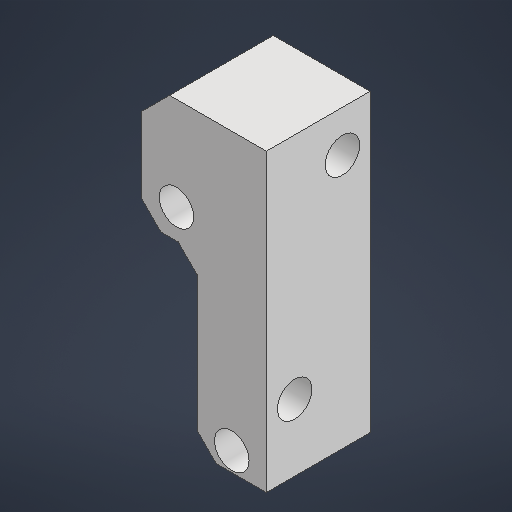
# Autodesk Inventor part: xy转接连杆
Saved by Autodesk Inventor 2025 (Build 290162000, 162)
## iProperties
Created: 2025-12-12
Part Number: xy转接连杆
Material: 常规
Document SubType Name: Modeling
Designer: HZD
Density: 1 g/cm^3
Appearance: 默认
Author: HZD
Autodesk Inventor part; units mm, degrees
ref_plane "YZ Plane" through (0, 0, 0) normal (1, 0, 0) x (0, 1, 0)
ref_plane "XZ Plane" through (0, 0, 0) normal (0, 1, 0) x (-1, 0, 0)
ref_plane "XY Plane" through (0, 0, 0) normal (0, 0, 1) x (1, 0, 0)
sketch "草图1" plane through (0, 0, 0) normal (0, 0, 1) x (1, 0, 0)
  line L0 (9, -20) -> (-9, -20)
  line L1 (-9, -20) -> (-9, 20)
  line L2 (-9, 20) -> (9, 20)
  line L3 (9, 20) -> (9, -20)
  line L4 (9, -20) -> (-9, 20) construction
  line L5 (-9, -20) -> (9, 20) construction
  circle A0 centre (-4, 6.5) radius 2.5
  circle A1 centre (4, -7.0033) radius 2.5
  circle A2 centre (-4, 6.5) radius 2.5 projected
  circle A3 centre (4, -7.0033) radius 2.5 projected
  line L6 (6, -3.0033) -> (9, -6.0033) projected
  line L7 (6, -3.0033) -> (4, -3.0033) projected
  line L8 (1, -0.0033) -> (4, -3.0033) projected
  line L9 (1, -0.0033) -> (1, 20.9967) projected
  line L10 (4, 23.9967) -> (1, 20.9967) projected
  line L11 (4, 23.9967) -> (6, 23.9967) projected
  line L12 (6, 26.9967) -> (6, 23.9967) projected
  line L13 (6, 26.9967) -> (-12, 26.9967) projected
  line L14 (-12, -24.0033) -> (-12, 26.9967) projected
  line L15 (9, -24.0033) -> (-12, -24.0033) projected
  line L16 (9, -24.0033) -> (9, -6.0033) projected
  point P0 (0, 0)
  dimension "d0" = 18
  dimension "d3" = 40
  dimension "d15" = 5
  dimension "d16" = 8
  dimension "d17" = 5
  dimension "d18" = 13.5
  dimension "d22" = 0
  constraints: 12 end point, 2 centre point, 2 midpoint, 2 parallel, 1 horizontal, 1 perpendicular
  measures "d0" distance of L1.end L2.end
  measures "d3" distance of L0.end L1.end
  measures "d15" distance from line of L3 A1.centre
  measures "d16" horizontal distance of A1.centre A0.centre
  measures "d17" distance from line of A0.centre L1
  measures "d18" distance from line of L2 A0.centre
  measures "d22" distance of A3.centre A1.centre
extrude "拉伸1" add sketch "草图1" along normal blind 15 contours L0 L1 L2 L9 L8 L7 L6 L3 | L6 L7 L8 L9 L2 L3
sketch "草图2" plane through (9, -20, 0) normal (1, 0, 0) x (0, 0, -1)
  circle A0 centre (-10.9079, 6.8983) radius 2.5
  circle A1 centre (-4, 34) radius 2.5
  line L0 (0, 0) -> (0, 40) projected
  line L1 (0, 40) -> (-15, 40) projected
  line L2 (0, 0) -> (-15, 0) projected
  point P0 (0, 20)
  dimension "d4" = 27.1017
  dimension "d5" = 4
  dimension "d6" = 6.9079
  dimension "d7" = 6
  dimension "d8" = 6.8983
  dimension "d9" = 5
  dimension "d10" = 5
  constraints: 2 centre point
  measures "d4" vertical distance of A0.centre A1.centre
  measures "d5" distance from line of L0 A1.centre
  measures "d6" horizontal distance of A1.centre A0.centre
  measures "d7" distance from line of L1 A1.centre
  measures "d8" distance from line of A0.centre L2
  measures "d9" diameter of A0
  measures "d10" diameter of A1
extrude "拉伸2" cut sketch "草图2" against normal blind 15
chamfer "倒角1" distance 4 angle 45 2 edges at (-9, 20, 7.5) (-9, -20, 7.5)
sketch "草图3" plane through (-9, -16, 0) normal (-1, 0, 0) x (0, 0, 1)
  point P0 (0, 16)
move faces "移动1" translate (0, -6, 0) faces at (-0.3333, -20, 5)
delete faces "删除1" heal yes whole lump no faces at (-2.3333, -22.6667, 5)
move faces "移动2" translate (0, -13, 0) faces at (6.4919, -6.8022, 5)
move faces "移动3" translate (0, 3.25, 0) faces at (-3, -26, 5)
sketch "草图4" plane through (-5, 20, 15) normal (0, 0, 1) x (1, 0, 0)
  line L0 (-4, -4) -> (-4, -42.75) projected
  line L1 (-4, -42.75) -> (14, -42.75) projected
  line L2 (-4, -17.75) -> (4, -17.75)
  line L3 (4, -17.75) -> (4, -42.75)
  line L4 (4, -42.75) -> (-4, -42.75)
  line L5 (-4, -42.75) -> (-4, -17.75)
  point P0 (5, -20)
  dimension "d32" = 8
  dimension "d33" = 25
  constraints: 8 end point, 2 parallel, 2 point on line, 1 horizontal, 1 perpendicular
  measures "d32" distance between parallel lines of L3 L0
  measures "d33" distance between parallel lines of L1 L2
extrude "拉伸3" cut sketch "草图4" against normal blind 20.5
chamfer "倒角2" distance 2.75 angle 45 3 edges at (-1, 2.25, 7.5) (-9, 2.25, 7.5) (-1, -22.75, 7.5)
